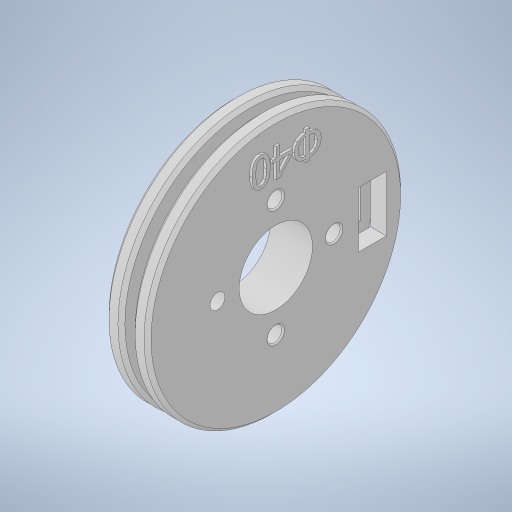
# Autodesk Inventor part: pully_elbow_40
Saved by Autodesk Inventor 2024 (Build 280153000, 153)
## iProperties
Created: 2025-06-10
Part Number: pully_elbow_40
Material: 一般
Document SubType Name: Modeling
Designer: HosodaLab2
Density: 1 g/cm^3
Appearance: 既定
Author: HosodaLab2
Autodesk Inventor part; units mm, degrees
ref_plane "YZ Plane" through (0, 0, 0) normal (1, 0, 0) x (0, 1, 0)
ref_plane "XZ Plane" through (0, 0, 0) normal (0, 1, 0) x (-1, 0, 0)
ref_plane "XY Plane" through (0, 0, 0) normal (0, 0, 1) x (1, 0, 0)
sketch "スケッチ1" plane through (0, 0, 0) normal (0, 1, 0) x (-1, 0, 0)
  circle A0 centre (0, 0) radius 20
  dimension "d0" = 40
  constraints: 1 centre point, 1 coincident
  measures "d0" diameter of A0
extrude "押し出し1" add sketch "スケッチ1" along normal blind 2.2
sketch "スケッチ2" plane through (0, 2.2, 0) normal (0, 1, 0) x (1, 0, 0)
  circle A0 centre (0, 0) radius 27.5
  line L0 (-2.1333, -14.239) -> (2.8564, -14.239) construction
  line L1 (2.8564, -14.239) -> (2.8564, -16.2928) construction
  line L2 (2.8564, -16.2928) -> (-2.1333, -16.2928) construction
  line L3 (-2.1333, -16.2928) -> (-2.1333, -14.239) construction
  dimension "d3" = 55
  constraints: 1 centre point, 1 coincident, 2 other
  measures "d3" diameter of A0
extrude "押し出し2" add sketch "スケッチ2" along normal blind 3.4
chamfer "面取り1" distance 0.75 angle 45 1 edges at (-27.5, 2.2, 0)
chamfer "面取り2" distance 0.75 angle 45 1 edges at (-27.5, 5.6, 0)
sketch "スケッチ3" plane through (0, 0, 0) normal (0, -1, 0) x (1, 0, 0)
  circle A0 centre (0, 0) radius 27.5
  dimension "d12" = 55
  constraints: 1 centre point, 1 coincident
  measures "d12" diameter of A0
extrude "押し出し3" add sketch "スケッチ3" along normal blind 3.4
chamfer "面取り3" distance 0.75 angle 45 1 edges at (-27.5, 0, 0)
chamfer "面取り4" distance 0.75 angle 45 1 edges at (-27.5, -3.4, 0)
sketch "スケッチ5" plane through (0, -3.4, 0) normal (0, -1, 0) x (1, 0, 0)
  circle A0 centre (0, 0) radius 12.5
  point P0 (0, -12.5)
  point P1 (0, 12.5)
  point P2 (-12.5, 0)
  point P3 (12.5, 0)
  dimension "d30" = 25
  constraints: 4 point on circle, 1 centre point, 1 coincident
  measures "d30" diameter of A0
hole "穴1" at (0, -3.4, -12.5) at (0, -3.4, 12.5) at (-12.5, -3.4, 0) at (12.5, -3.4, 0) direction (0, 1, 0) diameter 3.2 end through all
fillet "フィレット1" radius 0.3 6 edges at (0, -3.4, -10.9) (-12.5, -3.4, 1.6) (0, -3.4, 14.1) (0, 5.6, -10.9) (-12.5, 5.6, 1.6) (0, 5.6, 14.1)
sketch "スケッチ6" plane through (0, 5.6, 0) normal (0, 1, 0) x (1, 0, 0)
  circle A0 centre (0, 0) radius 3.15
  line L0 (0, 3.15) -> (39.8758, 3.15)
  circle A1 centre (0, 0) radius 40 projected
  line L1 (0, -3.15) -> (39.8758, -3.15)
  dimension "d39" = 6.3
  constraints: 4 end point, 4 point on circle, 1 centre point, 1 coincident, 1 horizontal, 1 parallel, 1 tangent
  measures "d39" diameter of A0
extrude "押し出し5" [suppressed]
chamfer "面取り7" [suppressed]
chamfer "面取り8" [suppressed]
chamfer "面取り9" [suppressed]
sketch "スケッチ7" plane through (0, 5.6, 0) normal (0, 1, 0) x (1, 0, 0)
  line L0 (-9.4901, -16.6138) -> (21.1536, -16.6138) construction
  line L1 (21.1536, -16.6138) -> (21.1536, -23.2125) construction
  line L2 (21.1536, -23.2125) -> (-9.4901, -23.2125) construction
  line L3 (-9.4901, -23.2125) -> (-9.4901, -16.6138) construction
  spline S0 degree 2 poles (-5.9458, -17.3355) (-5.3674, -17.3454) (-4.4084, -17.7309) (-4.092, -18.0522) knots 0 0 0 1 2 2 2
  spline S1 degree 2 poles (-4.092, -18.0522) (-3.8004, -18.3538) (-3.4791, -19.1991) (-3.4791, -19.7428) knots 0 0 0 1 2 2 2
  spline S2 degree 2 poles (-3.4791, -19.7428) (-3.4791, -20.3113) (-3.8251, -21.1863) (-4.1316, -21.4829) knots 0 0 0 1 2 2 2
  spline S3 degree 2 poles (-4.1316, -21.4829) (-4.4628, -21.8091) (-5.4317, -22.17) (-5.9458, -22.1799) knots 0 0 0 1 2 2 2
  line L4 (-5.9458, -22.1799) -> (-5.9458, -22.8868)
  line L5 (-5.9458, -22.8868) -> (-6.7565, -22.8868)
  line L6 (-6.7565, -22.8868) -> (-6.7565, -22.1799)
  spline S4 degree 2 poles (-6.7565, -22.1799) (-7.2706, -22.1651) (-8.2345, -21.8289) (-8.5756, -21.4928) knots 0 0 0 1 2 2 2
  spline S5 degree 2 poles (-8.5756, -21.4928) (-8.8821, -21.1912) (-9.2232, -20.3064) (-9.2232, -19.7428) knots 0 0 0 1 2 2 2
  spline S6 degree 2 poles (-9.2232, -19.7428) (-9.2232, -19.209) (-8.8969, -18.3637) (-8.6003, -18.0572) knots 0 0 0 1 2 2 2
  spline S7 degree 2 poles (-8.6003, -18.0572) (-8.2839, -17.7309) (-7.3348, -17.3503) (-6.7565, -17.3355) knots 0 0 0 1 2 2 2
  line L7 (-6.7565, -17.3355) -> (-6.7565, -16.6879)
  line L8 (-6.7565, -16.6879) -> (-5.9458, -16.6879)
  line L9 (-5.9458, -16.6879) -> (-5.9458, -17.3355)
  spline S8 degree 2 poles (-5.9458, -21.5669) (-5.575, -21.557) (-5.0016, -21.3346) (-4.8138, -21.1467) knots 0 0 0 1 2 2 2
  spline S9 degree 2 poles (-4.8138, -21.1467) (-4.5617, -20.8996) (-4.3244, -20.1927) (-4.3244, -19.7082) knots 0 0 0 1 2 2 2
  spline S10 degree 2 poles (-4.3244, -19.7082) (-4.3244, -19.3029) (-4.5518, -18.6356) (-4.7792, -18.4032) knots 0 0 0 1 2 2 2
  spline S11 degree 2 poles (-4.7792, -18.4032) (-4.9917, -18.1808) (-5.5553, -17.9682) (-5.9458, -17.9583) knots 0 0 0 1 2 2 2
  line L10 (-5.9458, -17.9583) -> (-5.9458, -21.5669)
  spline S12 degree 2 poles (-6.7565, -17.9583) (-7.147, -17.9633) (-7.7105, -18.1857) (-7.9231, -18.4032) knots 0 0 0 1 2 2 2
  spline S13 degree 2 poles (-7.9231, -18.4032) (-8.1505, -18.6306) (-8.3779, -19.3128) (-8.3779, -19.7082) knots 0 0 0 1 2 2 2
  spline S14 degree 2 poles (-8.3779, -19.7082) (-8.3779, -20.1927) (-8.1406, -20.9045) (-7.8885, -21.1467) knots 0 0 0 1 2 2 2
  spline S15 degree 2 poles (-7.8885, -21.1467) (-7.7006, -21.3247) (-7.1272, -21.562) (-6.7565, -21.5669) knots 0 0 0 1 2 2 2
  line L11 (-6.7565, -21.5669) -> (-6.7565, -17.9583)
  line L12 (1.1577, -20.7414) -> (0.431, -20.7414)
  line L13 (0.431, -20.7414) -> (0.431, -22.8373)
  line L14 (0.431, -22.8373) -> (-0.3549, -22.8373)
  line L15 (-0.3549, -22.8373) -> (-0.3549, -20.7414)
  line L16 (-0.3549, -20.7414) -> (-3.049, -20.7414)
  line L17 (-3.049, -20.7414) -> (-3.049, -19.8813)
  line L18 (-3.049, -19.8813) -> (-0.3203, -16.7373)
  line L19 (-0.3203, -16.7373) -> (0.431, -16.7373)
  line L20 (0.431, -16.7373) -> (0.431, -20.0839)
  line L21 (0.431, -20.0839) -> (1.1577, -20.0839)
  line L22 (1.1577, -20.0839) -> (1.1577, -20.7414)
  line L23 (-0.3549, -20.0839) -> (-0.3549, -17.7013)
  line L24 (-0.3549, -17.7013) -> (-2.4064, -20.0839)
  line L25 (-2.4064, -20.0839) -> (-0.3549, -20.0839)
  spline S16 degree 2 poles (5.6067, -19.7873) (5.6067, -21.4285) (4.6526, -22.9659) (3.659, -22.9659) knots 0 0 0 1 2 2 2
  spline S17 degree 2 poles (3.659, -22.9659) (2.6506, -22.9659) (1.7064, -21.3988) (1.7064, -19.7923) knots 0 0 0 1 2 2 2
  spline S18 degree 2 poles (1.7064, -19.7923) (1.7064, -18.1412) (2.6605, -16.6138) (3.659, -16.6138) knots 0 0 0 1 2 2 2
  spline S19 degree 2 poles (3.659, -16.6138) (4.6625, -16.6138) (5.6067, -18.1956) (5.6067, -19.7873) knots 0 0 0 1 2 2 2
  spline S20 degree 2 poles (4.5587, -21.646) (4.6773, -21.3445) (4.7762, -20.4151) (4.7762, -19.7873) knots 0 0 0 1 2 2 2
  spline S21 degree 2 poles (4.7762, -19.7873) (4.7762, -19.1595) (4.6773, -18.2352) (4.5537, -17.9237) knots 0 0 0 1 2 2 2
  spline S22 degree 2 poles (4.5537, -17.9237) (4.4302, -17.6123) (4.0001, -17.291) (3.659, -17.291) knots 0 0 0 1 2 2 2
  spline S23 degree 2 poles (3.659, -17.291) (3.3179, -17.291) (2.878, -17.6123) (2.7494, -17.9336) knots 0 0 0 1 2 2 2
  spline S24 degree 2 poles (2.7494, -17.9336) (2.6259, -18.245) (2.5369, -19.1941) (2.5369, -19.7923) knots 0 0 0 1 2 2 2
  spline S25 degree 2 poles (2.5369, -19.7923) (2.5369, -20.4349) (2.616, -21.295) (2.7445, -21.6312) knots 0 0 0 1 2 2 2
  spline S26 degree 2 poles (2.7445, -21.6312) (2.8631, -21.9475) (3.3031, -22.2886) (3.659, -22.2886) knots 0 0 0 1 2 2 2
  spline S27 degree 2 poles (3.659, -22.2886) (3.9951, -22.2886) (4.4351, -21.9673) (4.5587, -21.646) knots 0 0 0 1 2 2 2
  point P0 (0, 0)
  constraints: 2 other
extrude "押し出し6" add sketch "スケッチ7" along normal blind 0.5
sketch "スケッチ8" plane through (0, 5.6, 0) normal (0, 1, 0) x (1, 0, 0)
  line L0 (-17.7, 6) -> (-23.7, 6)
  line L1 (-23.7, 6) -> (-23.7, -6)
  line L2 (-23.7, -6) -> (-17.7, -6)
  line L3 (-17.7, -6) -> (-17.7, 6)
  arc A0 (-20, 0) -> (-20, 0) centre (0, 0) ccw projected
  point P0 (-20.7, -6)
  point P1 (-20.7, 6)
  dimension "d53" = 12
  dimension "d54" = 6
  dimension "d55" = 17.7
  constraints: 8 end point, 2 midpoint, 2 parallel, 1 horizontal, 1 perpendicular
  measures "d53" distance of point (-20.7, -6) point (-20.7, 6)
  measures "d54" distance between parallel lines of L1 L3
  measures "d55" distance from line of point (0, 0) L3
extrude "押し出し7" cut sketch "スケッチ8" against normal blind 7.5 contours L3 L2 A0 L0 | A0 L2 L1 L0 picked at (-18.4323, -0.6759)
sketch "スケッチ9" plane through (0, 5.6, 0) normal (0, 1, 0) x (1, 0, 0)
  point P0 (0, 0)
  point P1 (0, 0)
  constraints: 1 coincident
hole "穴2" at (0, 5.6, 0) direction (0, -1, 0) diameter 15.7 end through all
